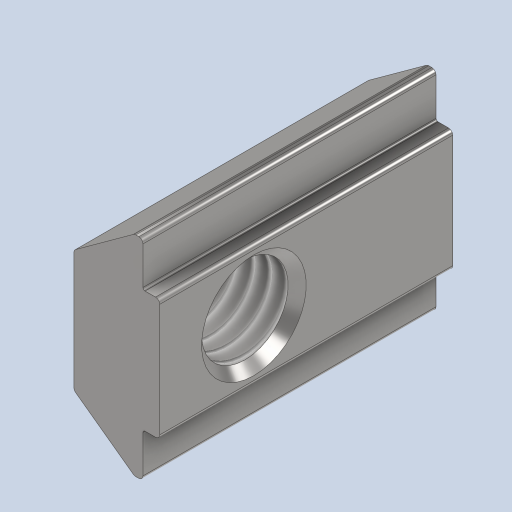
# Autodesk Inventor part: HNTU5-5
Saved by Autodesk Inventor 2023 (Build 270158000, 158)
## iProperties
Category: PARTsolutions
Company: MISUMI
Created: 2024-11-20
Part Number: HNTU5-5
Material: ステンレス鋼
Catalog Web Link: www.cadenas.de
Description: HNTU5, HNTUV5, HNTUZ5, SHNTU5-Pre-Assembly Insertion Nuts For HFS5 Series Aluminum Extrusions 20, 25, 40 Square
Vendor: MISUMI
Document SubType Name: Modeling
Designer: psAdmin
Manufacturer: MISUMI
Mass: 3.07994 g
Surface Area: 4.53089 cm^2
Volume: 0.384992 cm^3
Density: 8 g/cm^3
Appearance: 半つや出し
PSOL_IDENT_0: {$CADENAS_DATA/23d-libs/misumi/metric/38_al_extrusions_blackets/nuts/hntu5.prj},179 {VTYP=3D},{NB=HN
PSOL_IDENT_1: TU5-5},{LINA=HNTU5-5},{NN=HNTU5, HNTUV5, HNTUZ5, SHNTU5},{DATE=16.05.2023 02:30:27},{GEOMDATE=05.11.
PSOL_IDENT_2: 2019 07:02:46},{VERSION=},{LINEID=10},{WBVAR=M},{WBNUMERIC=M}  {NB=HNTU5-5},{LINA=HNTU5-5},{KT=DUMMY
PSOL_IDENT_3: },{PN=HNTU5-5},{TYPE=HNTU5},{TS=1010 Carbon Steel Equivalent},{M=5},{MALG=3, 4, 5},{T=4.1},{L1=4.5},
PSOL_IDENT_4: {A=5.800},{B=10},{E=3.3},{L=14},{M1=3.5},{L2=3.5}
NB: HNTU5-5
NN: HNTU5, HNTUV5, HNTUZ5, SHNTU5
NT: Pre-Assembly Insertion Nuts For HFS5 Series Aluminum Extrusions 20, 25, 40 Square
NBSYN: $PN.
LINA: HNTU5-5
CATALOG: Misumi
PN: HNTU5-5
TS: 1010 Carbon Steel Equivalent
M: 5
T: 4.1
L1: 4.5
SUPPLIER: MISUMI
ARTICLENO: HNTU5-5
BOMINFO: HNTU5-5
CREATOR: CADENAS GmbH
Title: HNTU5-5
Author: Cadenas PARTsolutions
Comments: Pre-Assembly Insertion Nuts For HFS5 Series Aluminum Extrusions 20, 25, 40 Square
Autodesk Inventor part; units mm, degrees
sketch "_____1" plane through (0, 0, 0) normal (0, 0, 1) x (1, 0, 0)
  line L0 (-4.1, 2.7981) -> (-4.1, -2.7981)
  arc A0 (-4.1, -2.7981) -> (-4.0176, -2.9599) centre (-3.9, -2.7981) ccw
  line L1 (-4.0176, -2.9599) -> (-1.2622, -4.9618)
  arc A1 (-1.2622, -4.9618) -> (-1.1446, -5) centre (-1.1446, -4.8) ccw
  line L2 (-1.1446, -5) -> (-1, -5)
  arc A2 (-1, -5) -> (-0.8, -4.8) centre (-1, -4.8) ccw
  line L3 (-0.8, -4.8) -> (-0.8, -3)
  arc A3 (-0.7, -2.9) -> (-0.8, -3) centre (-0.7, -3) ccw
  line L4 (-0.7, -2.9) -> (-0.2, -2.9)
  arc A4 (-0.2, -2.9) -> (0, -2.7) centre (-0.2, -2.7) ccw
  line L5 (0, -2.7) -> (0, 2.7)
  arc A5 (0, 2.7) -> (-0.2, 2.9) centre (-0.2, 2.7) ccw
  line L6 (-0.2, 2.9) -> (-0.7, 2.9)
  arc A6 (-0.8, 3) -> (-0.7, 2.9) centre (-0.7, 3) ccw
  line L7 (-0.8, 3) -> (-0.8, 4.8)
  arc A7 (-0.8, 4.8) -> (-1, 5) centre (-1, 4.8) ccw
  line L8 (-1, 5) -> (-1.1446, 5)
  arc A8 (-1.1446, 5) -> (-1.2622, 4.9618) centre (-1.1446, 4.8) ccw
  line L9 (-1.2622, 4.9618) -> (-4.0176, 2.9599)
  arc A9 (-4.0176, 2.9599) -> (-4.1, 2.7981) centre (-3.9, 2.7981) ccw
  constraints: 20 end point, 20 point on circle, 10 centre point
extrude "Extrusion1" add sketch "_____1" against normal blind 14
sketch "_____2" plane through (0, 0, -4.5) normal (0, 0, 1) x (1, 0, 0)
  line L0 (0, 0) -> (-4.1, 0)
  line L1 (-4.1, 0) -> (-4.1, 2.5)
  line L2 (-4.1, 2.5) -> (-3.667, 2.067)
  line L3 (-3.667, 2.067) -> (-0.433, 2.067)
  line L4 (-0.433, 2.067) -> (0, 2.5)
  line L5 (0, 2.5) -> (0, 0)
  line L6 (0, 0) -> (-4.1, 0)
  constraints: 14 end point
revolve "Revolution1" cut sketch "_____2" angle 360 about axis through (0, 0, -4.5) along (1, 0, 0)
thread "Thread1" size "M5x0.8" class "6H" standard "ISO Metric profile" full length
sketch "_____3" plane through (0, 0, -10.5) normal (0, 0, 1) x (1, 0, 0)
  line L0 (-3.05, 0) -> (-4.8, 0)
  line L1 (-4.8, 0) -> (-4.8, 1.75)
  line L2 (-4.8, 1.75) -> (-3.05, 1.75)
  line L3 (-3.05, 1.75) -> (-3.05, 0)
  line L4 (-3.05, 0) -> (-4.8, 0)
  constraints: 10 end point
revolve "Revolution2" cut sketch "_____3" angle 360 about axis through (-3.05, 0, -10.5) along (1, 0, 0)
sketch "_____4" plane through (0, 0, -10.5) normal (0, 0, 1) x (1, 0, 0)
  line L0 (-3.05, 1.75) -> (-3.05, -1.75)
  arc A0 (-3.05, 1.75) -> (-3.05, -1.75) centre (-3.05, 0) ccw
  line L1 (-3.05, 1.75) -> (-3.05, -1.75)
  constraints: 4 end point, 2 point on circle, 1 centre point
revolve "Revolution3" add sketch "_____4" angle 360 about axis through (-3.05, 1.75, -10.5) along (0, 1, 0)
ref_plane "to_blackets_XY" through (0, 0, -4.5) normal (1, 0, 0) x (0, 0, -1)
ref_plane "to_blackets_YZ" through (0, 0, -4.5) normal (0, 0, -1) x (0, 1, 0)
ref_plane "to_blackets_ZX" through (0, 0, -4.5) normal (0, 1, 0) x (1, 0, 0)
ref_plane "to_bolt_XY" through (-4.1, 0, -4.5) normal (1, 0, 0) x (0, 0, -1)
ref_plane "to_bolt_YZ" through (-4.1, 0, -4.5) normal (0, 0, -1) x (0, 1, 0)
ref_plane "to_bolt_ZX" through (-4.1, 0, -4.5) normal (0, 1, 0) x (1, 0, 0)
ref_plane "to_frames_XY" through (-0.8, 0, -4.5) normal (1, 0, 0) x (0, 0, -1)
ref_plane "to_frames_YZ" through (-0.8, 0, -4.5) normal (0, 0, -1) x (0, 1, 0)
ref_plane "to_frames_ZX" through (-0.8, 0, -4.5) normal (0, 1, 0) x (1, 0, 0)
body "Solid1"
